Autodesk Inventor part; units mm, degrees
(part 3 of 3)
  line L1804 (8.9446, 15.621) -> (8.9973, 15.6325)
  line L1805 (8.9973, 15.6325) -> (9.0532, 15.6531)
  line L1806 (9.0532, 15.6531) -> (9.112, 15.6831)
  line L1807 (9.112, 15.6831) -> (9.1734, 15.7224)
  line L1808 (9.1734, 15.7224) -> (9.237, 15.7712)
  line L1809 (9.237, 15.7712) -> (9.3692, 15.8979)
  line L1810 (9.3692, 15.8979) -> (9.5056, 16.0637)
  line L1811 (9.5056, 16.0637) -> (9.6033, 16.2048)
  line L1812 (9.6033, 16.2048) -> (9.7094, 16.3443)
  line L1813 (9.7094, 16.3443) -> (9.9128, 16.5707)
  line L1814 (9.9128, 16.5707) -> (10.0559, 16.7119)
  line L1815 (10.0559, 16.7119) -> (10.231, 16.8707)
  line L1816 (10.231, 16.8707) -> (10.4364, 17.042)
  line L1817 (10.4364, 17.042) -> (10.6756, 17.225)
  line L1818 (10.6756, 17.225) -> (10.9491, 17.4167)
  line L1819 (10.9491, 17.4167) -> (11.257, 17.6139)
  line L1820 (11.257, 17.6139) -> (11.603, 17.8155)
  line L1821 (11.603, 17.8155) -> (11.985, 18.0173)
  line L1822 (11.985, 18.0173) -> (12.3629, 18.1977)
  arc A39 (13.4867, 17.3813) -> (12.3629, 18.1977) centre (0, 0) ccw
  line L1823 (13.4867, 17.3813) -> (13.4319, 16.9661)
  line L1824 (13.4319, 16.9661) -> (13.3581, 16.5404)
  line L1825 (13.3581, 16.5404) -> (13.2732, 16.149)
  line L1826 (13.2732, 16.149) -> (13.1808, 15.7953)
  line L1827 (13.1808, 15.7953) -> (13.083, 15.4759)
  line L1828 (13.083, 15.4759) -> (12.9829, 15.1918)
  line L1829 (12.9829, 15.1918) -> (12.8835, 14.9436)
  line L1830 (12.8835, 14.9436) -> (12.7865, 14.728)
  line L1831 (12.7865, 14.728) -> (12.6964, 14.5482)
  line L1832 (12.6964, 14.5482) -> (12.544, 14.2849)
  line L1833 (12.544, 14.2849) -> (12.4441, 14.1408)
  line L1834 (12.4441, 14.1408) -> (12.3401, 14.0043)
  line L1835 (12.3401, 14.0043) -> (12.2245, 13.8234)
  line L1836 (12.2245, 13.8234) -> (12.1449, 13.6585)
  line L1837 (12.1449, 13.6585) -> (12.1181, 13.5829)
  line L1838 (12.1181, 13.5829) -> (12.0997, 13.5124)
  line L1839 (12.0997, 13.5124) -> (12.0894, 13.4472)
  line L1840 (12.0894, 13.4472) -> (12.0871, 13.3876)
  line L1841 (12.0871, 13.3876) -> (12.0924, 13.334)
  line L1842 (12.0924, 13.334) -> (12.1051, 13.2865)
  line L1843 (12.1051, 13.2865) -> (12.125, 13.2456)
  line L1844 (12.125, 13.2456) -> (12.1596, 13.2041)
  line L1845 (12.1596, 13.2041) -> (12.3906, 12.9876)
  line L1846 (12.3906, 12.9876) -> (12.6926, 12.6926)
  line L1847 (12.6926, 12.6926) -> (12.9876, 12.3906)
  line L1848 (12.9876, 12.3906) -> (13.2041, 12.1596)
  line L1849 (13.2041, 12.1596) -> (13.2456, 12.125)
  line L1850 (13.2456, 12.125) -> (13.2865, 12.1051)
  line L1851 (13.2865, 12.1051) -> (13.334, 12.0924)
  line L1852 (13.334, 12.0924) -> (13.3876, 12.0871)
  line L1853 (13.3876, 12.0871) -> (13.4472, 12.0894)
  line L1854 (13.4472, 12.0894) -> (13.5124, 12.0997)
  line L1855 (13.5124, 12.0997) -> (13.5829, 12.1181)
  line L1856 (13.5829, 12.1181) -> (13.6585, 12.1449)
  line L1857 (13.6585, 12.1449) -> (13.8234, 12.2245)
  line L1858 (13.8234, 12.2245) -> (14.0043, 12.3401)
  line L1859 (14.0043, 12.3401) -> (14.1408, 12.4441)
  line L1860 (14.1408, 12.4441) -> (14.2849, 12.544)
  line L1861 (14.2849, 12.544) -> (14.5482, 12.6964)
  line L1862 (14.5482, 12.6964) -> (14.728, 12.7865)
  line L1863 (14.728, 12.7865) -> (14.9436, 12.8835)
  line L1864 (14.9436, 12.8835) -> (15.1918, 12.9829)
  line L1865 (15.1918, 12.9829) -> (15.4759, 13.083)
  line L1866 (15.4759, 13.083) -> (15.7953, 13.1808)
  line L1867 (15.7953, 13.1808) -> (16.149, 13.2732)
  line L1868 (16.149, 13.2732) -> (16.5404, 13.3581)
  line L1869 (16.5404, 13.3581) -> (16.9661, 13.4319)
  line L1870 (16.9661, 13.4319) -> (17.3813, 13.4867)
  arc A40 (18.1977, 12.3629) -> (17.3813, 13.4867) centre (0, 0) ccw
  line L1871 (18.1977, 12.3629) -> (18.0173, 11.985)
  line L1872 (18.0173, 11.985) -> (17.8155, 11.603)
  line L1873 (17.8155, 11.603) -> (17.6139, 11.257)
  line L1874 (17.6139, 11.257) -> (17.4167, 10.9491)
  line L1875 (17.4167, 10.9491) -> (17.225, 10.6756)
  line L1876 (17.225, 10.6756) -> (17.042, 10.4364)
  line L1877 (17.042, 10.4364) -> (16.8707, 10.231)
  line L1878 (16.8707, 10.231) -> (16.7119, 10.0559)
  line L1879 (16.7119, 10.0559) -> (16.5707, 9.9128)
  line L1880 (16.5707, 9.9128) -> (16.3443, 9.7094)
  line L1881 (16.3443, 9.7094) -> (16.2048, 9.6033)
  line L1882 (16.2048, 9.6033) -> (16.0637, 9.5056)
  line L1883 (16.0637, 9.5056) -> (15.8979, 9.3692)
  line L1884 (15.8979, 9.3692) -> (15.7712, 9.237)
  line L1885 (15.7712, 9.237) -> (15.7224, 9.1734)
  line L1886 (15.7224, 9.1734) -> (15.6831, 9.112)
  line L1887 (15.6831, 9.112) -> (15.6531, 9.0532)
  line L1888 (15.6531, 9.0532) -> (15.6325, 8.9973)
  line L1889 (15.6325, 8.9973) -> (15.621, 8.9446)
  line L1890 (15.621, 8.9446) -> (15.6184, 8.8956)
  line L1891 (15.6184, 8.8956) -> (15.6247, 8.8505)
  line L1892 (15.6247, 8.8505) -> (15.6447, 8.8003)
  line L1893 (15.6447, 8.8003) -> (15.7975, 8.5231)
  line L1894 (15.7975, 8.5231) -> (15.9936, 8.1491)
  line L1895 (15.9936, 8.1491) -> (16.1809, 7.7707)
  line L1896 (16.1809, 7.7707) -> (16.3153, 7.4841)
  line L1897 (16.3153, 7.4841) -> (16.3442, 7.4385)
  line L1898 (16.3442, 7.4385) -> (16.3769, 7.4069)
  line L1899 (16.3769, 7.4069) -> (16.4181, 7.3801)
  line L1900 (16.4181, 7.3801) -> (16.4675, 7.3585)
  line L1901 (16.4675, 7.3585) -> (16.5249, 7.3423)
  line L1902 (16.5249, 7.3423) -> (16.5901, 7.3319)
  line L1903 (16.5901, 7.3319) -> (16.6629, 7.3277)
  line L1904 (16.6629, 7.3277) -> (16.743, 7.3298)
  line L1905 (16.743, 7.3298) -> (16.9244, 7.3546)
  line L1906 (16.9244, 7.3546) -> (17.1322, 7.4085)
  line L1907 (17.1322, 7.4085) -> (17.2942, 7.4653)
  line L1908 (17.2942, 7.4653) -> (17.462, 7.5158)
  line L1909 (17.462, 7.5158) -> (17.7596, 7.5794)
  line L1910 (17.7596, 7.5794) -> (17.9584, 7.6095)
  line L1911 (17.9584, 7.6095) -> (18.1934, 7.6351)
  line L1912 (18.1934, 7.6351) -> (18.4602, 7.6529)
  line L1913 (18.4602, 7.6529) -> (18.7613, 7.6604)
  line L1914 (18.7613, 7.6604) -> (19.0953, 7.6547)
  line L1915 (19.0953, 7.6547) -> (19.4602, 7.6332)
  line L1916 (19.4602, 7.6332) -> (19.8587, 7.593)
  line L1917 (19.8587, 7.593) -> (20.2864, 7.5317)
  line L1918 (20.2864, 7.5317) -> (20.6982, 7.4555)
  arc A41 (21.1274, 6.1345) -> (20.6982, 7.4555) centre (0, 0) ccw
  line L1919 (21.1274, 6.1345) -> (20.839, 5.8308)
  point P0 (21.1274, 6.1345)
  point P1 (20.6982, 7.4555)
  point P2 (18.1977, 12.3629)
  point P3 (17.3813, 13.4867)
  point P4 (13.4867, 17.3813)
  point P5 (12.3629, 18.1977)
  point P6 (7.4555, 20.6982)
  point P7 (6.1345, 21.1274)
  point P8 (0.6945, 21.989)
  point P9 (-0.6945, 21.989)
  point P10 (-6.1345, 21.1274)
  point P11 (-7.4555, 20.6982)
  point P12 (-12.3629, 18.1977)
  point P13 (-13.4867, 17.3813)
  point P14 (-17.3813, 13.4867)
  point P15 (-18.1977, 12.3629)
  point P16 (-20.6982, 7.4555)
  point P17 (-21.1274, 6.1345)
  point P18 (-21.989, 0.6945)
  point P19 (-21.989, -0.6945)
  point P20 (-21.1274, -6.1345)
  point P21 (-20.6982, -7.4555)
  point P22 (-18.1977, -12.3629)
  point P23 (-17.3813, -13.4867)
  point P24 (-13.4867, -17.3813)
  point P25 (-12.3629, -18.1977)
  point P26 (-7.4555, -20.6982)
  point P27 (-6.1345, -21.1274)
  point P28 (-0.6945, -21.989)
  point P29 (0.6945, -21.989)
  point P30 (6.1345, -21.1274)
  point P31 (7.4555, -20.6982)
  point P32 (12.3629, -18.1977)
  point P33 (13.4867, -17.3813)
  point P34 (17.3813, -13.4867)
  point P35 (18.1977, -12.3629)
  point P36 (20.6982, -7.4555)
  point P37 (21.1274, -6.1345)
  point P38 (21.989, -0.6945)
  point P39 (21.989, 0.6945)
  dimension "d2" = 26.5
  constraints: 3840 end point, 80 point on circle, 42 centre point
  measures "d2" diameter of A0
extrude "Extrusion1" add sketch "Sketch1" along normal blind 15
body "Solid1"
